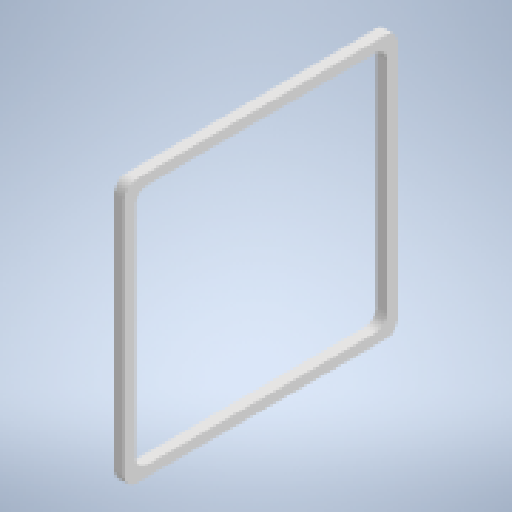
# Autodesk Inventor part: Pés
Saved by Autodesk Inventor 2025.2 (Build 292293000, 293)
## iProperties
Created: 2025-04-02
Part Number: Pés
Material: Genérico
Document SubType Name: Sheet Metal
Designer: kenay
Density: 1 g/cm^3
Sheet Metal Rule: Padrão_mm
Appearance: Padrão
Author: kenay
Autodesk Inventor part; units mm, degrees
sketch "Esboço1" plane through (0, 0, 0) normal (1, 0, 0) x (0, 1, 0)
  line L0 (-340, -390) -> (340, -390)
  line L1 (375, -355) -> (375, 355)
  line L2 (340, 390) -> (-340, 390)
  line L3 (-375, 355) -> (-375, -355)
  line L4 (-375, -390) -> (375, 390) construction
  line L5 (375, -390) -> (-375, 390) construction
  line L6 (-310, -358.8) -> (310, -358.8)
  line L7 (345, -323.8) -> (345, 323.8)
  line L8 (310, 358.8) -> (-310, 358.8)
  line L9 (-345, 323.8) -> (-345, -323.8)
  line L10 (-345, -358.8) -> (345, 358.8) construction
  line L11 (345, -358.8) -> (-345, 358.8) construction
  arc A0 (345, 323.8) -> (310, 358.8) centre (310, 323.8) ccw
  arc A1 (375, 355) -> (340, 390) centre (340, 355) ccw
  arc A2 (340, -390) -> (375, -355) centre (340, -355) ccw
  arc A3 (310, -358.8) -> (345, -323.8) centre (310, -323.8) ccw
  arc A4 (-310, 358.8) -> (-345, 323.8) centre (-310, 323.8) ccw
  arc A5 (-345, -323.8) -> (-310, -358.8) centre (-310, -323.8) ccw
  arc A6 (-375, -355) -> (-340, -390) centre (-340, -355) ccw
  arc A7 (-340, 390) -> (-375, 355) centre (-340, 355) ccw
  point P0 (0, 0)
  dimension "d0" = 780
  dimension "d1" = 750
  dimension "d2" = 30
  dimension "d3" = 35
  dimension "d4" = 35
  dimension "d5" = 35
  constraints: 24 end point, 17 point on line, 16 point on circle, 16 tangent, 8 centre point, 5 equal radius, 4 midpoint, 4 parallel, 2 horizontal, 2 perpendicular
  measures "d0" distance between parallel lines of L0 L2
  measures "d1" distance of L4.end L5.end
  measures "d2" distance between parallel lines of L1 L7
  measures "d3" radius of A0
  measures "d4" radius of A1
  measures "d5" radius of A2
extrude "Extrusão1" add sketch "Esboço1" along normal mid plane 30
equation "\"Raio_vergadura\" = Espessura"
equation "\"Largura_alívio_de_vergadura\" = Espessura"
equation "\"Profundidade_alívio_de_vergadura\" = 0.5 * Espessura"
equation "\"Tamanho_alívio_de_dobra\" = 4 * Espessura"
equation "\"Remanescente_mínimo\" = 2 * Espessura"
equation "\"Raiodetransição\" = Raio_vergadura"
equation "\"Tamanho_de_raio_de_Jacobi\" = Raio_vergadura"
equation "\"TamanhoFolga\" = Espessura"
equation "\"Espessura\" = 0.5"
